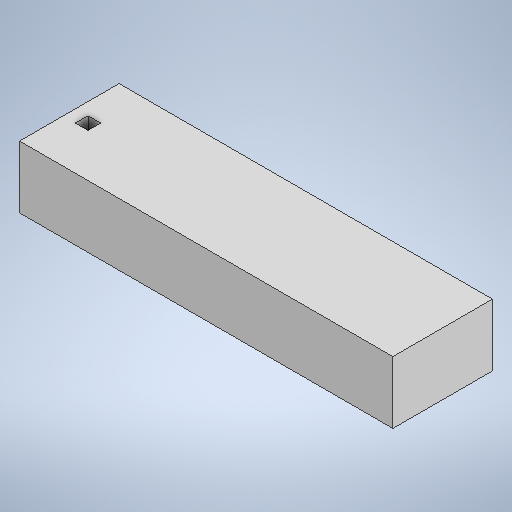
# Autodesk Inventor part: basketball post
Saved by Autodesk Inventor 2026.1 (Build 301233020, 233B)
## iProperties
Created: 2026-01-04
Part Number: basketball post
Material: Generic
Document SubType Name: Modeling
Designer: aa992
Density: 1 g/cm^3
Appearance: Default
Author: aa992
Autodesk Inventor part; units mm, degrees
ref_plane "YZ Plane" through (0, 0, 0) normal (1, 0, 0) x (0, 1, 0)
ref_plane "XZ Plane" through (0, 0, 0) normal (0, 1, 0) x (-1, 0, 0)
ref_plane "XY Plane" through (0, 0, 0) normal (0, 0, 1) x (1, 0, 0)
sketch "Sketch1" plane through (0, 0, 0) normal (0, 1, 0) x (-1, 0, 0)
  line L0 (150, 40) -> (-150, 40)
  line L1 (-150, 40) -> (-150, -40)
  line L2 (-150, -40) -> (150, -40)
  line L3 (150, -40) -> (150, 40)
  point P0 (0, 0)
  dimension "d0" = 300
  dimension "d1" = 80
  dimension "d2" = 40
  dimension "d3" = 150
  constraints: 8 end point, 2 parallel, 1 horizontal, 1 perpendicular
  measures "d0" distance of L1.end L2.end
  measures "d1" distance of L2.end L0.start
  measures "d2" distance from line of point (0, 0) L2
  measures "d3" distance from line of point (0, 0) L3
extrude "Extrusion1" add sketch "Sketch1" along normal blind 50
sketch "Sketch2" plane through (0, 50, 0) normal (0, 1, 0) x (1, 0, 0)
  line L0 (-140.1, -5.1) -> (-129.9, -5.1)
  line L1 (-129.9, -5.1) -> (-129.9, 5.1)
  line L2 (-129.9, 5.1) -> (-140.1, 5.1)
  line L3 (-140.1, 5.1) -> (-140.1, -5.1)
  line L4 (-150, 40) -> (-150, -40) projected
  line L5 (-150, -40) -> (150, -40) projected
  point P0 (0, 0)
  dimension "d6" = 10.2
  dimension "d7" = 10.2
  dimension "d8" = 9.9
  dimension "d9" = 34.9
  constraints: 8 end point, 2 parallel, 1 horizontal, 1 perpendicular
  measures "d6" distance of L2.end L1.end
  measures "d7" distance of L2.end L0.start
  measures "d8" distance between parallel lines of L3 L4
  measures "d9" distance between parallel lines of L5 L0
extrude "Extrusion2" cut sketch "Sketch2" against normal blind 20
body "Solid1"
